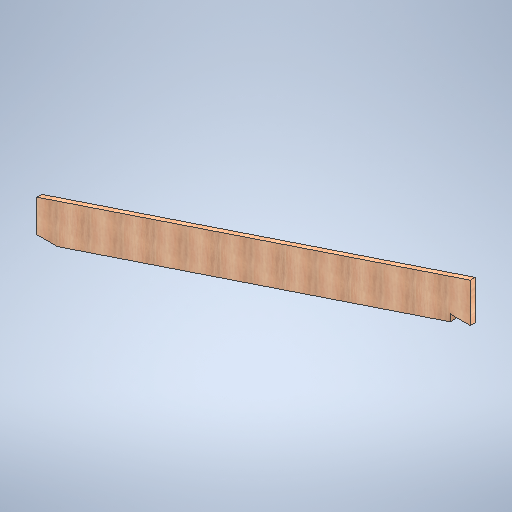
# Autodesk Inventor part: Rafter
Saved by Autodesk Inventor 2025 (Build 290162010, 162A)
## iProperties
Created: 2024-09-15
Part Number: Rafter
Material: Wood (Birch)
Document SubType Name: Modeling
Designer: Tom
Density: 0.55 g/cm^3
Appearance: Birch - Natural Polished
Author: Tom
Autodesk Inventor part; units mm, degrees
ref_plane "YZ Plane" through (0, 0, 0) normal (1, 0, 0) x (0, 1, 0)
ref_plane "XZ Plane" through (0, 0, 0) normal (0, 1, 0) x (-1, 0, 0)
ref_plane "XY Plane" through (0, 0, 0) normal (0, 0, 1) x (1, 0, 0)
sketch "Sketch1" plane through (0, 0, 0) normal (0, 0, 1) x (1, 0, 0)
  line L0 (0, 0) -> (3230.5625, 1079.5)
  line L1 (3230.5625, 1387.4762) -> (-161.925, 253.8686)
  line L2 (0, 0) -> (-161.925, 0)
  line L3 (-161.925, 0) -> (-161.925, 253.8686)
  line L4 (-161.925, 253.8686) -> (1498.726, 808.779)
  line L5 (3230.5625, 1079.5) -> (3073.4, 1079.5)
  line L6 (3073.4, 1079.5) -> (3073.4, 1026.9838)
  line L7 (3230.5625, 1079.5) -> (3230.5625, 1387.4762)
  line L8 (-139.7, 0) -> (-139.7, 261.2951)
  line L9 (3213.1, 1079.5) -> (3213.1, 1381.641)
  dimension "d5" = 292.1
  dimension "d12" = 161.925
  dimension "d13" = 157.1625
  dimension "d17" = 139.7
  dimension "d18" = 139.7
  dimension "d19" = 3352.8
  dimension "d20" = 1079.5
  constraints: 20 end point, 5 point on line, 4 vertical, 2 coincident, 2 horizontal, 1 collinear, 1 perpendicular
  measures "d5" distance between parallel lines of L1 L0
  measures "d12" distance of L0.start L2.end
  measures "d13" distance of L0.end L5.end
  measures "d17" distance from line of L8 point (0, 0)
  measures "d18" distance from line of L9 L5.end
  measures "d19" distance between parallel lines of L8 L9
  measures "d20" vertical distance of L9.start point (0, 0)
extrude "Extrusion1" add sketch "Sketch1" along normal blind 38.1 contours L2 L8 L1 L9 L5 L6 L0 | L2 L3 L1 L8 | L5 L9 L1 L7
body "Solid1"
